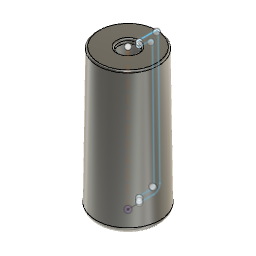
Kurbelgriff für Bürotisch ESB v12 (Autodesk Fusion 360 design; units mm, degrees)
Autodesk Fusion 360 part; units mm, degrees
ref_plane "Arbeitsebene11" through (0, 0, 3) normal (0, 0, 1) x (1, 0, 0)
sketch "Skizze34" plane through (0, 0, 3) normal (0, 0, 1) x (1, 0, 0)
  line L0 (0, 0) -> (0, 3) construction
  line L1 (0, 3.0015, 0.5015) -> (0, 3.0038, 1.3014)
  line L2 (0, 3.5038, 1.8) -> (0, 7.6485, 1.8)
  line L3 (0, 0, 0) -> (0, 0, 44) construction
  line L4 (0, 3.5069, 44) -> (0, 8.9068, 44)
  line L5 (0, 3.0069, 43.4932) -> (0, 3.0178, 42.6933)
  line L6 (0, 3.5178, 42.2002) -> (0, 7.1311, 42.2002)
  line L7 (0, 7.631, 41.7067) -> (0, 8.1484, 2.3066)
  line L8 (0, 3.5015) -> (0, 7.9725)
  line L9 (0, 9.4067, 43.5068) -> (0, 9.9724, 2.0273)
  arc A0 through (0, 9.9724, 2.0273) (0, 9.3964, 0.5955) (0, 7.9725, 0)
  arc A1 through (0, 7.6485, 1.8) (0, 8.0043, 1.9488) (0, 8.1484, 2.3066)
  arc A2 through (0, 3.0038, 1.3014) (0, 3.1507, 1.6541) (0, 3.5038, 1.8)
  arc A3 through (0, 3.5015, 0) (0, 3.1474, 0.147) (0, 3.0015, 0.5015)
  arc A4 through (0, 3.5038, 1.8) (0, 3.1507, 1.6541) (0, 3.0038, 1.3014)
  arc A5 through (0, 3.5015, 0) (0, 3.1474, 0.147) (0, 3.0015, 0.5015)
  arc A6 through (0, 3.0178, 42.6933) (0, 3.1666, 42.3442) (0, 3.5178, 42.2002)
  arc A7 through (0, 3.5069, 44) (0, 3.1509, 43.8511) (0, 3.0069, 43.4932)
  arc A8 through (0, 7.631, 41.7067) (0, 7.4823, 42.056) (0, 7.1311, 42.2002)
  arc A9 through (0, 9.4067, 43.5068) (0, 9.2579, 43.856) (0, 8.9068, 44)
  dimension "d120" = 3
  dimension "d123" = 44
  dimension "d131" = 2
  dimension "d133" = 0.5
  dimension "d134" = 0.5
  dimension "d135" = 0.5
  dimension "d136" = 0.5
  dimension "d137" = 0.5
  dimension "d138" = 0.5
  dimension "d139" = 0.5
  dimension "d140" = 0.5
  constraint coincident L0.start origin
  constraint vertical L0
  constraint coincident L0.end L8
  measures "d120" distance of L0.start L0.end
  measures "d123" distance of L0.start origin
revolve "Drehen2" add sketch "Skizze34" angle 360 about axis through (0, 0, 3) along (0, 0, 1) contours L1 L2 L4 L5 L6 L7 L8 L9 A0 A1 A2 A3 A4 A5 A6 A7 A8 A9 in plane through (0, 0, 3) normal (1, 0, 0)
named bodies: "Schwarzer Kunstoff Kurbelgriff (1)"
